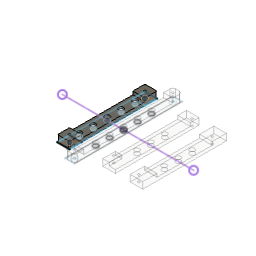
DIN Rail Mounts for Boards v6 (Autodesk Fusion 360 design; units mm, degrees)
Autodesk Fusion 360 part; units mm, degrees
sketch "Sketch1" plane through (0, 0, 0) normal (0, 0, 1) x (1, 0, 0) in component "CCM Dual Ethernet v2.a"
  circle A0 centre (0, 45) radius 0.95
  circle A1 centre (0, 0) radius 2.25
  line L0 (-56, 0) -> (64, 0) construction
  circle A2 centre (0, -45) radius 0.95
  line L1 (-4.25, 49.25) -> (4.25, 49.25)
  line L2 (4.25, 49.25) -> (4.25, -49.25)
  line L3 (4.25, -49.25) -> (-4.25, -49.25)
  line L4 (-4.25, -49.25) -> (-4.25, 49.25)
  circle A3 centre (0, -25.5) radius 2.25
  circle A4 centre (0, -12.75) radius 2.25
  circle A5 centre (0, 12.75) radius 2.25
  circle A6 centre (0, 25.5) radius 2.25
  dimension "d3" = 1.9
  dimension "d4" = 4.5
  dimension "d5" = 45
  dimension "d6" = 4.25
  dimension "d8" = 4.25
  dimension "d9" = 4.25
  dimension "d10" = 4.25
  dimension "d14" = 0
  dimension "d15" = 12.75
  constraint coincident A1.centre origin
  constraint horizontal L0
  constraint symmetric A0 L0 A2
  constraint horizontal L1
  constraint perpendicular L1 L2
  constraint parallel L1 L3
  constraint parallel L2 L4
  measures "d3" diameter of A0
  measures "d4" diameter of A1
  measures "d5" distance of A0.centre A1.centre
  measures "d6" distance of L2 A1.centre
  measures "d8" distance of A1.centre L4
  measures "d9" distance of A0.centre L1
  measures "d10" distance of A2.centre L3
extrude "Extrude1" add sketch "Sketch1" along normal blind 3 makes body 1 in component "CCM Dual Ethernet v2.a"
sketch "Sketch2" plane through (0, 0, 3) normal (0, 0, 1) x (-1, 0, 0) in component "CCM Dual Ethernet v2.a"
  circle A0 centre (0, -25.5) radius 2.25
  circle A1 centre (0, -12.75) radius 2.25
  circle A2 centre (0, 12.75) radius 2.25
  circle A3 centre (0, 0) radius 2.25
  circle A4 centre (0, -45) radius 0.95
  circle A5 centre (0, 45) radius 0.95
  circle A6 centre (0, 25.5) radius 2.25
  line L0 (4.25, 49.25) -> (-4.25, 49.25)
  line L1 (-4.25, 49.25) -> (-4.25, -49.25)
  line L2 (-4.25, -49.25) -> (4.25, -49.25)
  line L3 (4.25, -49.25) -> (4.25, 49.25)
  line L4 (4.25, -49.25) -> (-4.25, -49.25)
  line L5 (-4.25, -49.25) -> (-4.25, -40.75)
  line L6 (-4.25, -40.75) -> (4.25, -40.75)
  line L7 (4.25, -40.75) -> (4.25, -49.25)
  line L8 (56, 0) -> (-64, 0)
  line L9 (4.25, 49.25) -> (-4.25, 49.25)
  line L10 (-4.25, 40.75) -> (4.25, 40.75)
  line L11 (-4.25, 49.25) -> (-4.25, 40.75)
  line L12 (4.25, 40.75) -> (4.25, 49.25)
  constraint horizontal L4
  constraint vertical L5
  constraint horizontal L6
  constraint vertical L7
  constraint coincident L1 L5.end
  constraint coincident L2.end L3.start
  constraint equal L4 L7
  constraint symmetric L2.end L8 L0.start
  constraint symmetric L1.end L8 L0.end
  constraint symmetric L5.end L8 L10.start
  constraint symmetric L6.end L8 L10.end
extrude "Extrude2" add sketch "Sketch2" along normal blind 4 contours L1 L2 L3 L4 L5 L6 L7 | L0 L1 L3 L9 L10 L11 L12 bodies 1 in component "CCM Dual Ethernet v2.a"
fillet "Fillet1" radius 2.5 4 edges at (4.25, -49.25, 3.5) (-4.25, -49.25, 3.5) (4.25, 49.25, 3.5) (-4.25, 49.25, 3.5) on bodies 1 in component "CCM Dual Ethernet v2.a"
copy_body "CutPasteBodies1" bodies 1 removing the originals makes body 2 in component "CCM Dual Ethernet v2.a"
sketch "Sketch1 (2)" plane through (0, 0, 0) normal (0, 0, 1) x (1, 0, 0) in component "LeftMount"
  line L0 (19.25, 38.25) -> (30.75, 38.25)
  line L1 (30.75, 38.25) -> (30.75, -38.25)
  line L2 (30.75, -38.25) -> (19.25, -38.25)
  line L3 (19.25, -38.25) -> (19.25, 38.25)
  line L4 (19.25, 38.25) -> (30.75, -38.25) construction
  line L5 (30.75, 38.25) -> (19.25, -38.25) construction
  line L6 (-56, 0) -> (64, 0)
  point P0 (25, 0)
  dimension "d24" = 11.5
  dimension "d25" = 76.5
  constraint horizontal L0
  constraint perpendicular L0 L1
  constraint parallel L0 L2
  constraint parallel L1 L3
  constraint coincident L4 P0
  constraint coincident L5 P0
  constraint coincident P0 L6
  measures "d24" distance of L1.end L2.end
  measures "d25" distance of L0.end L1.end
extrude "Extrude1'" add sketch "Sketch1 (2)" along normal blind 3 separate body makes body 3 in component "LeftMount"
sketch "Sketch2 (2)" plane through (0, 0, 3) normal (0, 0, 1) x (-1, 0, 0) in component "LeftMount"
  line L0 (-19.25, 38.25) -> (-30.75, 38.25)
  line L1 (-30.75, 38.25) -> (-30.75, -38.25)
  line L2 (-30.75, -38.25) -> (-19.25, -38.25)
  line L3 (-19.25, -38.25) -> (-19.25, 38.25)
  line L4 (-19.25, -38.25) -> (-30.75, -38.25)
  line L5 (-30.75, -38.25) -> (-30.75, -30.25)
  line L6 (-30.75, -30.25) -> (-19.25, -30.25)
  line L7 (-19.25, -30.25) -> (-19.25, -38.25)
  line L8 (-19.25, 38.25) -> (-25.05, 38.25)
  line L9 (-25.05, 38.25) -> (-25.05, 26.75)
  line L10 (-25.05, 26.75) -> (-19.25, 26.75)
  line L11 (-19.25, 26.75) -> (-19.25, 38.25)
  dimension "d28" = 8
  dimension "d29" = 11.5
  dimension "d32" = 5.8
  constraint horizontal L4
  constraint vertical L5
  constraint horizontal L6
  constraint vertical L7
  constraint coincident L2 L3.start
  constraint horizontal L8
  constraint vertical L9
  constraint horizontal L10
  constraint vertical L11
  constraint coincident L0.start L3.end
  constraint coincident L3 L6.end
  measures "d28" distance of L2.end L6.end
  measures "d29" distance of L0.start L10.end
  measures "d32" distance of L0.start L8.end
extrude "Extrude2'" add sketch "Sketch2 (2)" along normal blind 3 contours L0 L3 L8 L9 L10 L11 | L1 L2 L3 L4 L5 L6 L7 bodies 3 in component "LeftMount"
sketch "Sketch3" plane through (0, 0, 6) normal (0, 0, 1) x (-1, 0, 0) in component "LeftMount"
  line L0 (-19.25, -30.25) -> (-30.75, -30.25)
  line L1 (-30.75, -30.25) -> (-30.75, -38.25)
  line L2 (-30.75, -38.25) -> (-19.25, -38.25)
  line L3 (-19.25, -38.25) -> (-19.25, -30.25)
  circle A0 centre (-28.25, -34.25) radius 0.95
  circle A1 centre (-21.75, 30.75) radius 0.95
  line L4 (-19.25, 26.75) -> (-19.25, 38.25)
  line L5 (-25.05, 26.75) -> (-19.25, 26.75)
  dimension "d33" = 1.9
  dimension "d35" = 9
  dimension "d36" = 4
  dimension "d37" = 1.9
  dimension "d38" = 2.5
  dimension "d39" = 4
  measures "d33" diameter of A0
  measures "d35" distance of L3 A0.centre
  measures "d36" distance of L0 A0.centre
  measures "d37" diameter of A1
  measures "d38" distance of A1.centre L4
  measures "d39" distance of A1.centre L5
extrude "Extrude3" cut sketch "Sketch3" against normal up to surface (6 mm away) contours A0 | A1 bodies 3 in component "LeftMount"
sketch "Sketch4" plane through (0, 0, 3) normal (0, 0, 1) x (-1, 0, 0) in component "LeftMount"
  line L0 (-30.75, -30.25) -> (-19.25, -30.25)
  line L1 (-19.25, -30.25) -> (-19.25, 26.75)
  line L2 (-19.25, 26.75) -> (-25.05, 26.75)
  line L3 (-25.05, 26.75) -> (-25.05, 38.25)
  line L4 (-25.05, 38.25) -> (-30.75, 38.25)
  line L5 (-30.75, 38.25) -> (-30.75, -30.25)
  circle A0 centre (-25, 0) radius 2.25
  circle A1 centre (-25, -12.75) radius 2.25
  circle A2 centre (-25, 12.75) radius 2.25
  dimension "d42" = 4.5
  dimension "d43" = 5.75
  dimension "d46" = 0
  dimension "d47" = 12.75
  measures "d42" diameter of A0
  measures "d43" distance of L1 A0.centre
extrude "Extrude4" cut sketch "Sketch4" against normal up to surface (3 mm away) contours A0 | A1 | A2 bodies 3 in component "LeftMount"
sketch "Sketch1 (3)" plane through (0, 0, 0) normal (0, 0, 1) x (1, 0, 0) in component "RightMount"
  line L0 (44.25, 38.25) -> (55.75, 38.25)
  line L1 (55.75, 38.25) -> (55.75, -38.25)
  line L2 (55.75, -38.25) -> (44.25, -38.25)
  line L3 (44.25, -38.25) -> (44.25, 38.25)
  line L4 (44.25, 38.25) -> (55.75, -38.25) construction
  line L5 (55.75, 38.25) -> (44.25, -38.25) construction
  line L6 (-56, 0) -> (64, 0)
  circle A0 centre (50, 0) radius 2.25
  circle A1 centre (50, -12.75) radius 2.25
  circle A2 centre (50, 12.75) radius 2.25
  point P0 (50, 0)
  dimension "d50" = 11.5
  dimension "d51" = 76.5
  dimension "d52" = 4.5
  dimension "d55" = 0
  dimension "d56" = 12.75
  constraint horizontal L0
  constraint perpendicular L0 L1
  constraint parallel L0 L2
  constraint parallel L1 L3
  constraint coincident L4 P0
  constraint coincident L5 P0
  constraint coincident P0 L6
  constraint coincident P0 A0.centre
  measures "d50" distance of L1.end L2.end
  measures "d51" distance of L0.end L1.end
  measures "d52" diameter of A0
extrude "Extrude1''" add sketch "Sketch1 (3)" along normal blind 3 separate body contours L0 L1 L3 L6 A0 | L1 L2 L3 L6 A0 makes body 4 in component "RightMount"
sketch "Sketch2 (3)" plane through (0, 0, 3) normal (0, 0, 1) x (-1, 0, 0) in component "RightMount"
  circle A0 centre (-50, 0) radius 2.25
  circle A1 centre (-50, 12.75) radius 2.25
  circle A2 centre (-50, -12.75) radius 2.25
  line L0 (-44.25, 38.25) -> (-55.75, 38.25)
  line L1 (-55.75, 38.25) -> (-55.75, -38.25)
  line L2 (-55.75, -38.25) -> (-44.25, -38.25)
  line L3 (-44.25, -38.25) -> (-44.25, 38.25)
  line L4 (-44.25, -38.25) -> (-55.75, -38.25)
  line L5 (-55.75, -38.25) -> (-55.75, -25.25)
  line L6 (-55.75, -25.25) -> (-44.25, -25.25)
  line L7 (-44.25, -25.25) -> (-44.25, -38.25)
  line L8 (-44.25, 38.25) -> (-55.75, 38.25)
  line L9 (-55.75, 38.25) -> (-55.75, 25.25)
  line L10 (-55.75, 25.25) -> (-44.25, 25.25)
  line L11 (-44.25, 25.25) -> (-44.25, 38.25)
  dimension "d59" = 13
  dimension "d60" = 13
  constraint horizontal L4
  constraint vertical L5
  constraint horizontal L6
  constraint vertical L7
  constraint coincident L2.end L3.start
  constraint horizontal L8
  constraint vertical L9
  constraint horizontal L10
  constraint vertical L11
  constraint coincident L0.start L3.end
  measures "d59" distance of L2.end L6.end
  measures "d60" distance of L0.start L10.end
extrude "Extrude2''" add sketch "Sketch2 (3)" along normal blind 3 contours L0 L1 L3 L8 L9 L10 L11 | L1 L2 L3 L4 L5 L6 L7 bodies 4 in component "RightMount"
sketch "Sketch3 (2)" plane through (0, 0, 6) normal (0, 0, 1) x (-1, 0, 0) in component "RightMount"
  line L0 (-44.25, -25.25) -> (-55.75, -25.25)
  line L1 (-55.75, -25.25) -> (-55.75, -38.25)
  line L2 (-55.75, -38.25) -> (-44.25, -38.25)
  line L3 (-44.25, -38.25) -> (-44.25, -25.25)
  circle A0 centre (-51.75, -29.25) radius 0.95
  circle A1 centre (-48.25, 34.25) radius 0.95
  line L4 (-44.25, 25.25) -> (-44.25, 38.25)
  line L5 (-44.25, 38.25) -> (-55.75, 38.25)
  dimension "d63" = 1.9
  dimension "d64" = 4
  dimension "d65" = 4
  dimension "d66" = 1.9
  dimension "d67" = 4
  dimension "d68" = 4
  measures "d63" diameter of A0
  measures "d64" distance of L1 A0.centre
  measures "d65" distance of L0 A0.centre
  measures "d66" diameter of A1
  measures "d67" distance of A1.centre L4
  measures "d68" distance of A1.centre L5
extrude "Extrude3'" cut sketch "Sketch3 (2)" against normal up to surface (6 mm away) contours A0 | A1 bodies 4 in component "RightMount"
sketch "Mount Base" plane through (0, 0, 0) normal (0, 0, 1) x (1, 0, 0) in component "Spring Fingers v2.a"
  circle A0 centre (-15, 34.5) radius 0.95
  line L0 (-56, 0) -> (64, 0)
  circle A1 centre (-15, -34.5) radius 0.95
  line L1 (-20.5, 40) -> (-9.5, 40)
  line L2 (-9.5, 40) -> (-9.5, -40)
  line L3 (-9.5, -40) -> (-20.5, -40)
  line L4 (-20.5, -40) -> (-20.5, 40)
  line L5 (-9.5, 29) -> (-20.5, 29)
  line L6 (-20.5, 29) -> (-20.5, 40)
  line L7 (-20.5, 40) -> (-9.5, 40)
  line L8 (-9.5, 40) -> (-9.5, 29)
  line L9 (-9.5, 29) -> (-20.5, 40) construction
  line L10 (-20.5, 29) -> (-9.5, 40) construction
  line L11 (-9.5, -40) -> (-20.5, -40)
  line L12 (-20.5, -40) -> (-20.5, -29)
  line L13 (-20.5, -29) -> (-9.5, -29)
  line L14 (-9.5, -29) -> (-9.5, -40)
  line L15 (-9.5, -40) -> (-20.5, -29) construction
  line L16 (-20.5, -40) -> (-9.5, -29) construction
  circle A2 centre (-15, 0) radius 2.25
  circle A3 centre (-15, -25.5) radius 2.25
  circle A4 centre (-15, -12.75) radius 2.25
  circle A5 centre (-15, 12.75) radius 2.25
  circle A6 centre (-15, 25.5) radius 2.25
  point P0 (-15, 34.5)
  point P1 (-15, -34.5)
  dimension "d71" = 1.9
  dimension "d72" = 34.5
  dimension "d73" = 5.5
  dimension "d74" = 5.5
  dimension "d75" = 5.5
  dimension "d76" = 5.5
  dimension "d82" = 4.5
  dimension "d85" = 0
  dimension "d86" = 12.75
  constraint symmetric A0 L0 A1
  constraint horizontal L1
  constraint vertical L2
  constraint horizontal L3
  constraint vertical L4
  constraint horizontal L5
  constraint perpendicular L5 L6
  constraint parallel L5 L7
  constraint parallel L6 L8
  constraint coincident L9 P0
  constraint coincident L10 P0
  constraint coincident L2 L5.start
  constraint coincident P0 A0.centre
  constraint horizontal L11
  constraint perpendicular L11 L12
  constraint parallel L11 L13
  constraint parallel L12 L14
  constraint coincident L15 P1
  constraint coincident L16 P1
  constraint coincident P1 A1.centre
  constraint coincident L0 A2.centre
  measures "d71" diameter of A0
  measures "d72" distance of P0 L0
  measures "d73" distance of P0 L1
  measures "d74" distance of P1 L3
  measures "d75" distance of P0 L4
  measures "d76" distance of P0 L2
  measures "d82" diameter of A2
extrude "Extrude1'''" add sketch "Mount Base" along normal blind 3 separate body contours L0 L2 L4 L5 A2 | L0 L2 L4 L13 A2 | L2 L3 L4 L11 L12 L13 L14 | L1 L2 L4 L5 L6 L7 L8 makes body 5 in component "Spring Fingers v2.a"
extrude "Extrude2'''" add sketch "Mount Base" along normal blind 6 contours L2 L3 L4 L11 L12 L13 L14 | L1 L2 L4 L5 L6 L7 L8 bodies 5 in component "Spring Fingers v2.a"
fillet "Fillet1'" radius 1 4 edges at (-9.5, -40, 3) (-20.5, -40, 3) (-9.5, 40, 3) (-20.5, 40, 3) on bodies 5 in component "Spring Fingers v2.a"
component "CCM Dual Ethernet v2.a" placed x (1, 0, 0) y (0, 1, 0) z (0, 0, 1) at (0, 0, 0)
component "Project Lab v3.e" placed x (1, 0, 0) y (0, 1, 0) z (0, 0, 1) at (0, 0, 0)
component "Spring Fingers v2.a" placed x (1, 0, 0) y (0, 1, 0) z (0, 0, 1) at (0, 0, 0)
component "LeftMount" placed x (1, 0, 0) y (0, 1, 0) z (0, 0, 1) at (0, 0, 0) in component "Project Lab v3.e"
component "RightMount" placed x (1, 0, 0) y (0, 1, 0) z (0, 0, 1) at (0, 0, 0) in component "Project Lab v3.e"
equation "PCBMountingHoleDiameter = 1.9 mm"
equation "DINMountingHoleDiameter = 4.5 mm"
equation "d3 = PCBMountingHoleDiameter"
equation "d4 = DINMountingHoleDiameter"
equation "d6 = ( DINMountingHoleDiameter / 2 ) + MinimumHoleToEdge"
equation "MinimumHoleToEdge = 2 mm"
equation "d8 = d6"
equation "d9 = d6"
equation "d10 = d6"
equation "MountThickness = 3 mm"
equation "d16 = MountThickness"
equation "d26 = MountThickness"
equation "d30 = MountThickness"
equation "d33 = PCBMountingHoleDiameter"
equation "d37 = PCBMountingHoleDiameter"
equation "d42 = DINMountingHoleDiameter"
equation "d43 = ( 11.5 / 2 ) * 1 mm"
equation "d52 = DINMountingHoleDiameter"
equation "d57 = MountThickness"
equation "d61 = MountThickness"
equation "d63 = PCBMountingHoleDiameter"
equation "d66 = PCBMountingHoleDiameter"
equation "d71 = PCBMountingHoleDiameter"
equation "d73 = DINMountingHoleDiameter + 1 mm"
equation "d74 = d73"
equation "d75 = d73"
equation "d76 = d73"
equation "d77 = MountThickness"
equation "d79 = 2 * MountThickness"
equation "d82 = DINMountingHoleDiameter"
